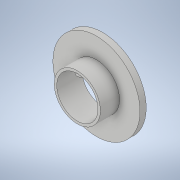
# Autodesk Inventor part: MotorFlexHub
Saved by Autodesk Inventor 2021 (Build 250183000, 183)
## iProperties
Created: 2020-09-16
Part Number: MotorFlexHub
Material: Generic
Document SubType Name: Modeling
Designer: PhotonUser
Density: 1 g/cm^3
Appearance: Default
Author: PhotonUser
Autodesk Inventor part; units mm, degrees
ref_plane "YZ Plane" through (0, 0, 0) normal (1, 0, 0) x (0, 1, 0)
ref_plane "XZ Plane" through (0, 0, 0) normal (0, 1, 0) x (-1, 0, 0)
ref_plane "XY Plane" through (0, 0, 0) normal (0, 0, 1) x (1, 0, 0)
sketch "Sketch1" plane through (0, 0, 0) normal (1, 0, 0) x (0, 1, 0)
  line L0 (0, 0) -> (24.892, 0)
  line L1 (24.892, 0) -> (24.892, -20.6502)
  line L2 (24.892, -20.6502) -> (47.0027, -20.6502)
  line L3 (47.0027, -20.6502) -> (47.0027, -27.3812)
  line L4 (47.0027, -27.3812) -> (0, -27.3812)
  line L5 (0, -27.3812) -> (0, 0)
  dimension "d1" = 24.892
  dimension "d2" = 20.6502
  dimension "d3" = 22.1107
  dimension "d4" = 6.731
  constraints: 12 end point, 3 perpendicular, 2 horizontal, 1 vertical
  measures "d1" distance of L0.start L0.end
  measures "d2" distance of L0.end L1.end
  measures "d3" distance of L1.end L2.end
  measures "d4" distance of L2.end L3.end
revolve "Revolution1" add sketch "Sketch1" angle 360 about axis through (0, 0, -27.3812) along (0, 0, 1)
sketch "Sketch2" plane through (0, 0, 0) normal (0, 0, 1) x (1, 0, 0)
  circle A0 centre (0, 0) radius 22.225
  dimension "d6" = 44.45
  constraints: 1 centre point, 1 coincident
  measures "d6" diameter of A0
extrude "Extrusion1" cut sketch "Sketch2" against normal blind 28.575
sketch "Sketch3" plane through (0, 0, 0) normal (0, 0, 1) x (1, 0, 0)
  circle A0 centre (0, 0) radius 22.225
  line L0 (-4.7625, 21.708736) -> (-4.7625, 19.551195)
  line L1 (-4.7625, 19.551195) -> (4.7625, 19.551195)
  line L2 (4.7625, 19.551195) -> (4.7625, 21.708736)
  arc A1 (4.7625, 21.701769) -> (-4.7625, 21.701769) centre (0, 0) ccw
  line L3 (0, 0) -> (0, 24.892)
  circle A2 centre (0, 0) radius 24.892
  point P0 (0, 22.218195)
  dimension "d10" = 9.525
  dimension "d12" = 2.667
  constraints: 8 end point, 5 point on circle, 3 point on line, 2 perpendicular, 2 vertical, 1 centre point, 1 coincident, 1 vertical alignment, 1 other
  measures "d10" distance between parallel lines of L2 L0
  measures "d12" distance from line of L1 point (0, 22.218)
sketch "Sketch3 outline for Extrusion2" plane through (0, 0, 0) normal (0, 0, 1) x (1, 0, 0)
  arc A0 (4.7625, 21.701769) -> (-4.7625, 21.701769) centre (0, 0) ccw
  line L0 (4.7625, 19.551195) -> (4.7625, 21.701769)
  line L1 (-4.7625, 19.551195) -> (4.7625, 19.551195)
  line L2 (-4.7625, 21.701769) -> (-4.7625, 19.551195)
extrude "Extrusion2" add sketch "Sketch3 outline for Extrusion2" against normal up to surface (27.3812 mm away)
sketch "Sketch4" plane through (-4.7625, 19.551195, 0) normal (0, -1, 0) x (1, 0, 0)
  line L0 (4.7625, 0) -> (4.7625, -4.7752)
  arc A0 (9.525, -5.123236) -> (0, -5.123236) centre (4.7625, -4.7752) ccw
  line L1 (9.525, 0) -> (0, 0)
  line L2 (4.7625, 0) -> (0, 0)
  line L3 (0, 0) -> (0, -4.427164)
  line L4 (0, 0) -> (0, -27.3812)
  line L5 (4.7625, 0) -> (9.5377, 0)
  line L6 (9.5377, 0) -> (9.525, -4.427164)
  line L7 (9.525, 0) -> (9.525, -27.3812)
  dimension "d15" = 4.7752
  constraints: 10 end point, 5 point on circle, 5 point on line, 1 centre point, 1 coincident, 1 horizontal, 1 tangent, 1 vertical
  measures "d15" distance of L0.start L0.end
extrude "Extrusion3" cut sketch "Sketch4" against normal up to surface contours A0 L3 L1 | A0 L1 L7
body "Solid1"
